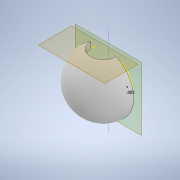
# Autodesk Inventor part: Head front
Saved by Autodesk Inventor 2020 (Build 240168000, 168)
## iProperties
Created: 2022-05-03
Part Number: Head front
Material: Generic
Document SubType Name: Modeling
Designer: Administrator
Density: 1 g/cm^3
Appearance: Default
Author: Administrator
Autodesk Inventor part; units mm, degrees
ref_plane "YZ Plane" through (0, 0, 0) normal (1, 0, 0) x (0, 1, 0)
ref_plane "XY Plane" through (0, 0, 0) normal (0, 0, 1) x (1, 0, 0)
sketch "Sketch1" plane through (0, 0, 0) normal (0, 0, 1) x (1, 0, 0)
  arc A0 (0, -8.6995) -> (0, 8.6995) centre (0, 0) ccw
  line L0 (0, 8.6995) -> (0, -8.6995)
  dimension "d0" = 17.399
  constraints: 2 end point, 2 point on circle, 1 centre point, 1 coincident, 1 vertical
  measures "d0" diameter of A0
revolve "Revolution1" add sketch "Sketch1" angle 180 about axis through (0, 8.6995, 0) along (0, -1, 0)
shell "Shell1" thickness 1.651 removed faces 2 at (4.2263, 0.0174, 0) at (-4.2263, 0.0174, 0)
ref_plane "Work Plane1" through (0, 8.6995, 0) normal (0, 1, 0) x (-1, 0, 0)
sketch "Sketch2" plane through (0, 8.6995, 0) normal (0, 1, 0) x (-1, 0, 0)
  circle A0 centre (0, 0) radius 3.683
  dimension "d4" = 7.366
  constraints: 1 centre point, 1 coincident
  measures "d4" diameter of A0
extrude "Extrusion1" cut sketch "Sketch2" against normal blind 5.08
ref_plane "Work Plane2" through (0, 0, -1.397) normal (0, 0, -1) x (-1, 0, 0)
sketch "Sketch3" plane through (0, 0, -1.397) normal (0, 0, -1) x (-1, 0, 0)
  circle A0 centre (-5.969, 0) radius 1.0795
  arc A1 (-3.683, 6.0097) -> (3.683, 6.0097) centre (0, 0) ccw projected
  line L0 (0, 12.9331) -> (0, -13.6064) construction
  circle A2 centre (5.969, 0) radius 1.0795
  dimension "d8" = 2.159
  constraints: 2 centre point, 2 end point, 1 horizontal alignment, 1 symmetric about line, 1 tangent, 1 vertical, 1 other
  measures "d8" diameter of A0
body "Solid1"
